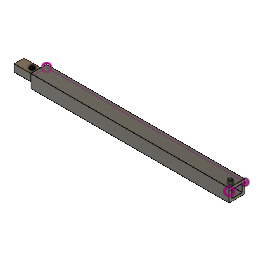
Half Tie Rod Type A (Autodesk Fusion 360 design; units mm, degrees)
Autodesk Fusion 360 part; units mm, degrees
note: some values were not read from the file. Set by a fixed rule: which sketch regions a step uses.
sketch "Sketch1" plane through (0, 0, 0) normal (0, 0, 1) x (1, 0, 0)
  line L0 (0, 0) -> (150, 0)
  line L1 (150, 0) -> (150, -12)
  line L2 (150, -12) -> (0, -12)
  line L3 (0, -12) -> (0, 0)
  dimension "d16" = 150
  dimension "d17" = 12
  constraint horizontal L0
  constraint vertical L1
  constraint horizontal L2
  constraint vertical L3
  constraint coincident L0.start L3.end
  measures "d16" distance of L0.start L0.end
  measures "d17" distance of L0.start L2.end
extrude "Extrude1" add sketch "Sketch1" along normal blind 10
sketch "Sketch3" plane through (0, 0, 0) normal (-1, 0, 0) x (0, -1, 0)
  line L0 (0, 0) -> (12, 0)
  line L1 (12, 0) -> (12, 10)
  line L2 (12, 10) -> (0, 10)
  line L3 (0, 10) -> (0, 0)
  line L4 (2.2, 7.8) -> (9.8, 7.8)
  line L5 (9.8, 7.8) -> (9.8, 2.2)
  line L6 (9.8, 2.2) -> (2.2, 2.2)
  line L7 (2.2, 2.2) -> (2.2, 7.8)
  dimension "d22" = 7.6
  dimension "d23" = 5.6
  dimension "d26" = 2.2
  dimension "d27" = 2.2
  constraint horizontal L4
  constraint vertical L5
  constraint horizontal L6
  constraint vertical L7
  measures "d22" distance of L4.start L4.end
  measures "d23" distance of L4.start L6.end
  measures "d26" distance of L3 L7
  measures "d27" distance of L2 L4
extrude "Extrude2" add sketch "Sketch3" along normal blind 15 contours L4 L5 L6 L7
sketch "Sketch4" plane through (150, 0, 0) normal (1, 0, 0) x (0, 1, 0)
  line L0 (-12, 0) -> (0, 0)
  line L1 (0, 0) -> (0, 10)
  line L2 (0, 10) -> (-12, 10)
  line L3 (-12, 10) -> (-12, 0)
  line L4 (-10, 8) -> (-2, 8)
  line L5 (-2, 8) -> (-2, 2)
  line L6 (-2, 2) -> (-10, 2)
  line L7 (-10, 2) -> (-10, 8)
  dimension "d30" = 6
  dimension "d31" = 8
  dimension "d34" = 2
  dimension "d35" = 2
  constraint horizontal L4
  constraint vertical L5
  constraint horizontal L6
  constraint vertical L7
  measures "d30" distance of L4.start L6.end
  measures "d31" distance of L4.start L4.end
  measures "d34" distance of L3 L7
  measures "d35" distance of L2 L4
extrude "Extrude3" cut sketch "Sketch4" against normal blind 15 contours L4 L5 L6 L7
sketch "Sketch5" plane through (0, 0, 7.8) normal (0, 0, 1) x (-1, 0, 0)
  line L0 (0, 2.2) -> (15, 2.2)
  line L1 (15, 2.2) -> (15, 9.8)
  line L2 (15, 9.8) -> (0, 9.8)
  circle A0 centre (5, 6) radius 1.5
  circle A1 centre (-145, 6) radius 1.5
  line L3 (-150, 12) -> (-150, 0)
  line L4 (-150, 0) -> (0, 0)
  line L5 (0, 9.8) -> (0, 2.2)
  dimension "d37" = 3
  dimension "d38" = 3
  dimension "d43" = 10
  dimension "d44" = 3.8
  dimension "d45" = 5
  dimension "d46" = 6
  measures "d37" diameter of A0
  measures "d38" diameter of A1
  measures "d43" distance of L1 A0.centre
  measures "d44" distance of L0 A0.centre
  measures "d45" distance of A1.centre L3
  measures "d46" distance of A1.centre L4
extrude "Extrude4" cut sketch "Sketch5" against normal blind 100 contours A0
extrude "Extrude5" cut sketch "Sketch5" along normal mid plane 200 contours A1
equation "main_length = 150 mm"
equation "height = 10 mm"
equation "dowel_edge_width = 7.6 mm"
equation "dowel_edge_length = 15 mm"
equation "length = 180 mm"
equation "edge_hole_radius = 1.5 mm"
equation "dowel_edge_hole_big_distance = 10 mm"
equation "dowel_edge_hole_small_distance = dowel_edge_width / 2"
equation "hollow_edge_length = 15 mm"
equation "hollow_edge_width = 8 mm"
equation "width = 12 mm"
equation "dowel_edge_height = 5.6 mm"
equation "hollow_edge_height = 6 mm"
equation "hollow_edge_hole_big_distance = 5 mm"
equation "hollow_edge_hole_small_distance = width / 2"
equation "d16 = main_length"
equation "d17 = width"
equation "d18 = height"
equation "dowel_edge_small_distance = ( width - dowel_edge_width ) / 2"
equation "dowel_edge_big_distance = ( height - dowel_edge_height ) / 2"
equation "d22 = dowel_edge_width"
equation "d23 = dowel_edge_height"
equation "d24 = dowel_edge_length"
equation "d26 = dowel_edge_big_distance"
equation "d27 = dowel_edge_small_distance"
equation "hollow_edge_small_distance = ( width - hollow_edge_width ) / 2"
equation "hollow_edge_big_distance = ( height - hollow_edge_height ) / 2"
equation "d30 = hollow_edge_height"
equation "d31 = hollow_edge_width"
equation "d32 = -hollow_edge_length"
equation "d34 = hollow_edge_big_distance"
equation "d35 = hollow_edge_small_distance"
equation "extra = 100 mm"
equation "d37 = edge_hole_radius * 2"
equation "d38 = edge_hole_radius * 2"
equation "d39 = -extra"
equation "d41 = extra"
equation "d43 = dowel_edge_hole_big_distance"
equation "d44 = dowel_edge_hole_small_distance"
equation "d45 = hollow_edge_hole_big_distance"
equation "d46 = hollow_edge_hole_small_distance"
